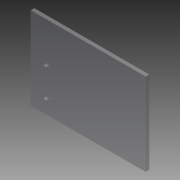
# Autodesk Inventor part: Polycarbonate Board Circuit Breaker
Saved by Autodesk Inventor 2014 (Build 180170000, 170)
## iProperties
Created: 2014-01-22
Part Number: Polycarbonate Board Circuit Breaker
Material: Polycarbonate, Clear
Document SubType Name: Modeling
Designer: Andrew Toennies
Mass: 17.1038 g
Surface Area: 99.4808 cm^2
Volume: 14.2532 cm^3
Density: 1.2 g/cm^3
Appearance: Polycarbonate - Clear
Author: Andrew Toennies
Autodesk Inventor part; units mm, degrees
ref_plane "YZ Plane" through (0, 0, 0) normal (1, 0, 0) x (0, 1, 0)
ref_plane "XZ Plane" through (0, 0, 0) normal (0, 1, 0) x (-1, 0, 0)
ref_plane "XY Plane" through (0, 0, 0) normal (0, 0, 1) x (1, 0, 0)
sketch "Sketch1" plane through (0, 0, 0) normal (0, 0, 1) x (1, 0, 0)
  line L0 (0, 0) -> (76.2, 0)
  line L1 (76.2, 0) -> (76.2, 73.025)
  line L2 (76.2, 73.025) -> (25.4, 73.025)
  line L3 (0, 50.8) -> (0, 0)
  circle A0 centre (12.7, 38.1) radius 2.0701
  circle A1 centre (12.7, 12.7) radius 2.0701
  line L4 (12.7, 38.1) -> (12.7, 12.7) construction
  line L5 (0, 50.8) -> (25.4, 50.8)
  line L6 (25.4, 50.8) -> (25.4, 73.025)
  dimension "d2" = 4.1402
  dimension "d3" = 4.1402
  dimension "d4" = 12.7
  dimension "d5" = 12.7
  dimension "d6" = 25.4
  dimension "d9" = 25.4
  dimension "d10" = 50.8
  dimension "d11" = 50.8
  dimension "d12" = 73.025
  constraints: 14 end point, 3 parallel, 3 perpendicular, 2 centre point, 1 horizontal
  measures "d2" diameter of A0
  measures "d3" diameter of A1
  measures "d4" distance between parallel lines of L3 L4
  measures "d5" distance from line of L0 L4.end
  measures "d6" distance of L4.start L4.end
  measures "d9" distance of L3.start L5.end
  measures "d10" distance between parallel lines of L0 L5
  measures "d11" distance of L1.end L2.end
  measures "d12" distance between parallel lines of L0 L2
extrude "Extrusion1" add sketch "Sketch1" along normal blind 3.175
body "Solid1"
